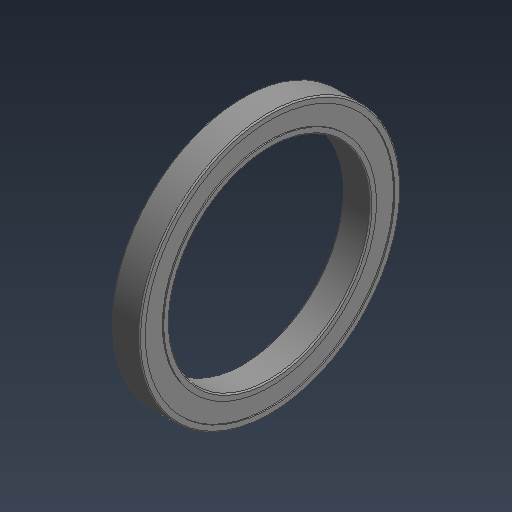
# Autodesk Inventor part: B6810ZZ
Saved by Autodesk Inventor 2021 (Build 250183000, 183)
## iProperties
Category: PARTsolutions
Company: MISUMI
Part Number: B6810ZZ
Material: 一般
Catalog Web Link: www.cadenas.de
Description: B6_ _ _ZZ, SB6_ _ _ZZ-Deep Groove Ball Bearings - Double Shield Type
Vendor: MISUMI
Document SubType Name: Modeling
Designer: partserver
Manufacturer: MISUMI
Mass: 8.94087 g
Surface Area: 53.7803 cm^2
Volume: 8.94087 cm^3
Density: 1 g/cm^3
Appearance: PSOLRGB-175-175-175
PSOL_IDENT_0: {$CADENAS_DATA\23d-libs\misumi\metric\12_bearing_holders\sb6010zz.prj},172 {VTYP=3D},{NB=B6810ZZ},{L
PSOL_IDENT_1: INA=B6810ZZ},{NN=B6_ _ _ZZ, SB6_ _ _ZZ},{DATE=22.10.2019 07:39:52},{GEOMDATE=22.10.2019 06:26:04},{V
PSOL_IDENT_2: ERSION=},{LINEID=410},{WBVAR=TS},{WBNUMERIC=}  {NB=B6810ZZ},{LINA=B6810ZZ},{KT=DUMMY},{PN=B6810ZZ},{
PSOL_IDENT_3: TS=},{TS1= '', 'Steel', 'S', 'Stainless Steel'},{MAT=52100 Bearing Steel},{BN=6810ZZ},{DD=50},{D=65}
PSOL_IDENT_4: ,{B=7},{RR=0.3},{CR=6.6},{COR=6.09},{CRS=6.6},{CRSS=5.61},{CORS=6.09},{CORSS=4.80},{DD1=0.00},{R1=0.
PSOL_IDENT_5: 00},{R2=0.0},{DSMIN=52.0},{DSMAX=52.50},{DS1=52.50},{DDHH=63.0},{R=0.3},{MASS=50},{MASS11=50},{AA=6.
PSOL_IDENT_6: 3560},{BB=1.5000},{CC=1.4500},{TYS=w/o Retaining Ring}
NB: B6810ZZ
NN: B6_ _ _ZZ, SB6_ _ _ZZ
NT: Deep Groove Ball Bearings - Double Shield Type
NBSYN: $PN.
LINA: B6810ZZ
CATALOG: Misumi
PN: B6810ZZ
TS: Steel
MAT: 52100 Bearing Steel
BN: 6810ZZ
DD: 50
D: 65
B: 7
RR: 0.3
CR: 6.6
COR: 6.09
DSMIN: 52
DSMAX: 52.5
DDHH: 63
R: 0.3
MASS: 50
SUPPLIER: MISUMI
ARTICLENO: B6810ZZ
BOMINFO: B6810ZZ
CREATOR: CADENAS GmbH
購入先: ミスミ
在庫数: 0.0
Title: B6810ZZ
Author: Cadenas PARTsolutions
Comments: Deep Groove Ball Bearings - Double Shield Type
Autodesk Inventor part; units mm, degrees
sketch "Sketch_1" plane through (0, 0, 0) normal (0, 0, 1) x (1, 0, 0)
  line L0 (7, 0) -> (0, 0)
  arc A0 (0, 25.3) -> (0.3, 25) centre (0.3, 25.3) ccw
  line L1 (0.3, 25) -> (6.7, 25)
  arc A1 (6.7, 25) -> (7, 25.3) centre (6.7, 25.3) ccw
  line L2 (7, 25.3) -> (7, 26.45)
  line L3 (7, 26.45) -> (6.678, 26.45)
  line L4 (6.678, 26.45) -> (6.678, 31)
  line L5 (6.678, 31) -> (7, 31)
  line L6 (7, 31) -> (7, 32.2)
  arc A2 (7, 32.2) -> (6.7, 32.5) centre (6.7, 32.2) ccw
  line L7 (6.7, 32.5) -> (0.3, 32.5)
  arc A3 (0.3, 32.5) -> (0, 32.2) centre (0.3, 32.2) ccw
  line L8 (0, 32.2) -> (0, 31)
  line L9 (0, 31) -> (0.322, 31)
  line L10 (0.322, 31) -> (0.322, 26.45)
  line L11 (0.322, 26.45) -> (0, 26.45)
  line L12 (0, 26.45) -> (0, 25.3)
  constraints: 26 end point, 8 point on circle, 4 centre point
revolve "Revolution1" add sketch "Sketch_1" angle 360 about axis through (7, 0, 0) along (1, 0, 0)
ref_plane "center_point_XY" through (3.5, 0, 0) normal (1, 0, 0) x (0, 0, -1)
ref_plane "center_point_YZ" through (3.5, 0, 0) normal (0, 0, -1) x (0, 1, 0)
ref_plane "center_point_ZX" through (3.5, 0, 0) normal (0, 1, 0) x (1, 0, 0)
ref_plane "to_housing_XY" through (0, 0, 0) normal (1, 0, 0) x (0, 0, -1)
ref_plane "to_housing_YZ" through (0, 0, 0) normal (0, 0, -1) x (0, 1, 0)
ref_plane "to_housing_ZX" through (0, 0, 0) normal (0, 1, 0) x (1, 0, 0)
ref_plane "to_ring_XY" through (6.356, 0, 0) normal (1, 0, 0) x (0, 0, -1)
ref_plane "to_ring_YZ" through (6.356, 0, 0) normal (0, 0, -1) x (0, 1, 0)
ref_plane "to_ring_ZX" through (6.356, 0, 0) normal (0, 1, 0) x (1, 0, 0)
body "Solid1"
